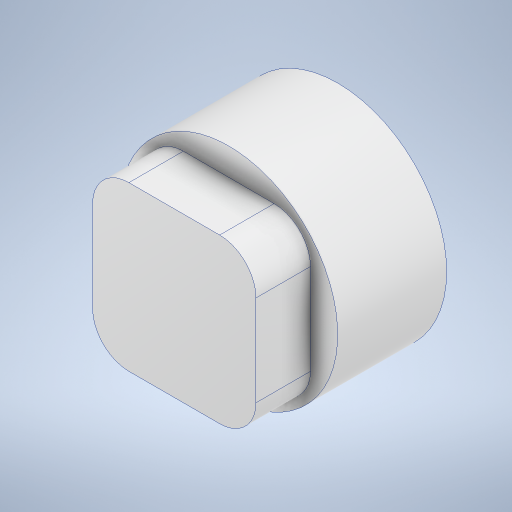
# Autodesk Inventor part: Nakrętka na belkę
Saved by Autodesk Inventor 2024 (Build 280153000, 153)
## iProperties
Created: 2024-04-13
Part Number: Nakrętka na belkę
Material: Aluminum 6061
Document SubType Name: Modeling
Designer: HP
Density: 2.7 g/cm^3
Appearance: Aluminum - Flat
Author: HP
Autodesk Inventor part; units mm, degrees
ref_plane "YZ Plane" through (0, 0, 0) normal (1, 0, 0) x (0, 1, 0)
ref_plane "XZ Plane" through (0, 0, 0) normal (0, 1, 0) x (-1, 0, 0)
ref_plane "XY Plane" through (0, 0, 0) normal (0, 0, 1) x (1, 0, 0)
sketch "Sketch1" plane through (0, 0, 0) normal (0, 0, 1) x (1, 0, 0)
  circle A0 centre (0, 0) radius 4
  circle A1 centre (0, 0) radius 6
  dimension "d0" = 8
  dimension "d1" = 12
  constraints: 2 centre point, 2 coincident
  measures "d0" diameter of A0
  measures "d1" diameter of A1
extrude "Extrusion1" add sketch "Sketch1" along normal blind 6
sketch "Sketch2" plane through (0, 0, 6) normal (0, 0, 1) x (1, 0, 0)
  line L0 (-4.5, -4.5) -> (4.5, -4.5)
  line L1 (4.5, -4.5) -> (4.5, 4.5)
  line L2 (4.5, 4.5) -> (-4.5, 4.5)
  line L3 (-4.5, 4.5) -> (-4.5, -4.5)
  line L4 (-4.5, -4.5) -> (4.5, 4.5) construction
  line L5 (4.5, -4.5) -> (-4.5, 4.5) construction
  point P0 (0, 0)
  dimension "d4" = 9
  dimension "d5" = 9
  constraints: 12 end point, 2 midpoint, 2 parallel, 1 horizontal, 1 perpendicular
  measures "d4" distance of L2.end L1.end
  measures "d5" distance of L1.end L0.end
extrude "Extrusion2" add sketch "Sketch2" along normal blind 3
fillet "Fillet1" radius 2 4 edges at (-4.5, -4.5, 7.5) (-4.5, 4.5, 7.5) (4.5, 4.5, 7.5) (4.5, -4.5, 7.5)
thread "Thread1" size "M8x1.25" class "6H" standard "ANSI Metric M Profile" length 6
body "Solid1"
